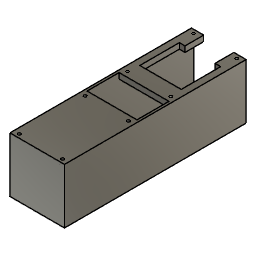
6_Cell_Lipo_Holder v3 (Autodesk Fusion 360 design; units mm, degrees)
Autodesk Fusion 360 part; units mm, degrees
sketch "Sketch1" plane through (0, 0, 0) normal (0, 1, 0) x (1, 0, 0)
  line L0 (26, -24.75) -> (-26, -24.75)
  line L1 (-26, -24.75) -> (-26, 24.75)
  line L2 (-26, 24.75) -> (26, 24.75)
  line L3 (26, 24.75) -> (26, -24.75)
  line L4 (26, -24.75) -> (-26, 24.75) construction
  line L5 (-26, -24.75) -> (26, 24.75) construction
  dimension "d1" = 52
  dimension "d2" = 49.5
  constraint horizontal L0
  constraint perpendicular L0 L1
  constraint parallel L0 L2
  constraint parallel L1 L3
  constraint coincident L4 origin
  constraint coincident L5 origin
  measures "d1" distance of L0.start L0.end
  measures "d2" distance of L0.start L2.end
extrude "Extrude1" add sketch "Sketch1" along normal blind 155 makes body 1
sketch "Sketch2" plane through (0, 0, 0) normal (0, -1, 0) x (1, 0, 0)
  line L0 (-26, -24.75) -> (26, -24.75)
  line L1 (26, -24.75) -> (26, 24.75)
  line L2 (26, 24.75) -> (-26, 24.75)
  line L3 (-26, 24.75) -> (-26, -24.75)
  line L4 (32, 30.75) -> (-32, 30.75)
  line L5 (-32, 30.75) -> (-32, -30.75)
  line L6 (-32, -30.75) -> (32, -30.75)
  line L7 (32, -30.75) -> (32, 30.75)
  line L8 (32, 30.75) -> (-32, -30.75) construction
  line L9 (-32, 30.75) -> (32, -30.75) construction
  dimension "d5" = 64
  dimension "d6" = 61.5
  constraint horizontal L4
  constraint perpendicular L4 L5
  constraint parallel L4 L6
  constraint parallel L5 L7
  constraint coincident L8 origin
  constraint coincident L9 origin
  measures "d5" distance of L4.start L4.end
  measures "d6" distance of L4.start L6.end
extrude "Extrude2" add sketch "Sketch2" against normal blind 193 separate body contours L0 L1 L2 L3 | L4 L5 L6 L7 makes body 2
sketch "Sketch3" plane through (0, 193, 0) normal (0, 1, 0) x (-1, 0, 0)
  line L0 (-32, 30.75) -> (-32, -30.75)
  line L1 (-32, -30.75) -> (32, -30.75)
  line L2 (32, -30.75) -> (32, 30.75)
  line L3 (32, 30.75) -> (-32, 30.75)
  line L4 (26, 24.75) -> (-26, 24.75)
  line L5 (-26, 24.75) -> (-26, -24.75)
  line L6 (-26, -24.75) -> (26, -24.75)
  line L7 (26, -24.75) -> (26, 24.75)
  line L8 (26, 24.75) -> (-26, -24.75) construction
  line L9 (-26, 24.75) -> (26, -24.75) construction
  dimension "d9" = 52
  dimension "d10" = 49.5
  constraint horizontal L4
  constraint perpendicular L4 L5
  constraint parallel L4 L6
  constraint parallel L5 L7
  constraint coincident L8 origin
  constraint coincident L9 origin
  measures "d9" distance of L4.start L4.end
  measures "d10" distance of L4.start L6.end
extrude "Extrude3" cut sketch "Sketch3" against normal blind 160 contours L4 L5 L6 L7 bodies 2
move_body "Move1" bodies 1 to x (1, 0, 0) y (0, 1, 0) z (0, 0, 1) at (0, 320, 0)
sketch "Sketch6" plane through (0, 0, 30.75) normal (0, 0, 1) x (-1, 0, 0)
  line L0 (32, 0) -> (-32, 0)
  line L1 (-32, 0) -> (-32, -193)
  line L2 (-32, -193) -> (32, -193)
  line L3 (32, -193) -> (32, 0)
  line L4 (0, 0) -> (0, -193)
  line L5 (32, -96.5) -> (-32, -96.5)
  circle A0 centre (-23, -4) radius 1.5
  circle A1 centre (23, -4) radius 1.5
  circle A2 centre (-23, -74) radius 1.5
  circle A3 centre (23, -74) radius 1.5
  circle A4 centre (-23, -119) radius 1.5
  circle A5 centre (23, -119) radius 1.5
  circle A6 centre (23, -189) radius 1.5
  circle A7 centre (-23, -189) radius 1.5
  line L6 (26, -79.5) -> (-26, -79.5)
  line L7 (-26, -79.5) -> (-26, -113.5)
  line L8 (-26, -113.5) -> (26, -113.5)
  line L9 (26, -113.5) -> (26, -79.5)
  line L10 (26, -79.5) -> (-26, -113.5) construction
  line L11 (-26, -79.5) -> (26, -113.5) construction
  line L12 (22, -131.0349) -> (-22, -131.0349)
  line L13 (-22, -131.0349) -> (-22, -173.0349)
  line L14 (-22, -173.0349) -> (22, -173.0349)
  line L15 (22, -173.0349) -> (22, -131.0349)
  line L16 (22, -131.0349) -> (-22, -173.0349) construction
  line L17 (-22, -131.0349) -> (22, -173.0349) construction
  point P0 (0, -96.5)
  point P1 (0, -152.0349)
  dimension "d45" = 3
  dimension "d46" = 3
  dimension "d47" = 3
  dimension "d48" = 3
  dimension "d49" = 3
  dimension "d50" = 3
  dimension "d51" = 3
  dimension "d52" = 3
  dimension "d53" = 23
  dimension "d54" = 23
  dimension "d55" = 23
  dimension "d56" = 23
  dimension "d57" = 22.5
  dimension "d58" = 22.5
  dimension "d59" = 70
  dimension "d60" = 70
  dimension "d89" = 52
  dimension "d90" = 34
  dimension "d101" = 44
  dimension "d102" = 42
  constraint coincident L4.start origin
  constraint midpoint L2 L4.end
  constraint midpoint L3 L5.start
  constraint midpoint L1 L5.end
  constraint symmetric L4 A0.centre A1.centre
  constraint symmetric L4 A2.centre A3.centre
  constraint symmetric L4 A4.centre A5.centre
  constraint symmetric L4 A6.centre A7.centre
  constraint horizontal L6
  constraint perpendicular L6 L7
  constraint parallel L6 L8
  constraint parallel L7 L9
  constraint coincident L10 P0
  constraint coincident L11 P0
  constraint midpoint L5 P0
  constraint horizontal L12
  constraint perpendicular L12 L13
  constraint parallel L12 L14
  constraint parallel L13 L15
  constraint coincident L16 P1
  constraint coincident L17 P1
  constraint coincident L4 P1
  measures "d45" diameter of A0
  measures "d46" diameter of A1
  measures "d47" diameter of A2
  measures "d48" diameter of A3
  measures "d49" diameter of A5
  measures "d50" diameter of A4
  measures "d51" diameter of A7
  measures "d52" diameter of A6
  measures "d53" distance of L4 A0.centre
  measures "d54" distance of L4 A2.centre
  measures "d55" distance of L4 A4.centre
  measures "d56" distance of L4 A7.centre
  measures "d57" distance of L5 A2.centre
  measures "d58" distance of L5 A4.centre
  measures "d59" distance of A0.centre A2.centre
  measures "d60" distance of A4.centre A7.centre
  measures "d89" distance of L6.start L6.end
  measures "d90" distance of L6.end L7.end
  measures "d101" distance of L12.start L12.end
  measures "d102" distance of L12.end L13.end
extrude "Extrude4" cut sketch "Sketch6" against normal blind 80 contours A0 | A1 | A2 | A3 | A4 | A5 | A6 | A7 bodies 2
sketch "Sketch7" plane through (0, 0, -30.75) normal (0, 0, -1) x (1, 0, 0)
  circle A0 centre (-23, -119) radius 1.5
  circle A1 centre (-23, -4) radius 1.5
  circle A2 centre (-23, -74) radius 1.5
  circle A3 centre (-23, -189) radius 1.5
  circle A4 centre (23, -119) radius 1.5
  circle A5 centre (23, -4) radius 1.5
  circle A6 centre (23, -74) radius 1.5
  circle A7 centre (23, -189) radius 1.5
  line L0 (32, 0) -> (-32, 0)
  line L1 (-32, 0) -> (-32, -193)
  line L2 (-32, -193) -> (32, -193)
  line L3 (32, -193) -> (32, 0)
  line L4 (20, -6) -> (26, -6)
  line L5 (26, -6) -> (26, -2)
  line L6 (26, -2) -> (20, -2)
  line L7 (20, -2) -> (20, -6)
  line L8 (20, -6) -> (26, -2) construction
  line L9 (26, -6) -> (20, -2) construction
  line L10 (-26, -6) -> (-20, -6)
  line L11 (-20, -6) -> (-20, -2)
  line L12 (-20, -2) -> (-26, -2)
  line L13 (-26, -2) -> (-26, -6)
  line L14 (-26, -6) -> (-20, -2) construction
  line L15 (-20, -6) -> (-26, -2) construction
  line L16 (20, -76) -> (26, -76)
  line L17 (26, -76) -> (26, -72)
  line L18 (26, -72) -> (20, -72)
  line L19 (20, -72) -> (20, -76)
  line L20 (20, -76) -> (26, -72) construction
  line L21 (26, -76) -> (20, -72) construction
  line L22 (-26, -76) -> (-20, -76)
  line L23 (-20, -76) -> (-20, -72)
  line L24 (-20, -72) -> (-26, -72)
  line L25 (-26, -72) -> (-26, -76)
  line L26 (-26, -76) -> (-20, -72) construction
  line L27 (-20, -76) -> (-26, -72) construction
  line L28 (-26, -121) -> (-20, -121)
  line L29 (-20, -121) -> (-20, -117)
  line L30 (-20, -117) -> (-26, -117)
  line L31 (-26, -117) -> (-26, -121)
  line L32 (-26, -121) -> (-20, -117) construction
  line L33 (-20, -121) -> (-26, -117) construction
  line L34 (20, -121) -> (26, -121)
  line L35 (26, -121) -> (26, -117)
  line L36 (26, -117) -> (20, -117)
  line L37 (20, -117) -> (20, -121)
  line L38 (20, -121) -> (26, -117) construction
  line L39 (26, -121) -> (20, -117) construction
  line L40 (20, -191) -> (26, -191)
  line L41 (26, -191) -> (26, -187)
  line L42 (26, -187) -> (20, -187)
  line L43 (20, -187) -> (20, -191)
  line L44 (20, -191) -> (26, -187) construction
  line L45 (26, -191) -> (20, -187) construction
  line L46 (-26, -191) -> (-20, -191)
  line L47 (-20, -191) -> (-20, -187)
  line L48 (-20, -187) -> (-26, -187)
  line L49 (-26, -187) -> (-26, -191)
  line L50 (-26, -191) -> (-20, -187) construction
  line L51 (-20, -191) -> (-26, -187) construction
  point P0 (23, -4)
  point P1 (-23, -4)
  point P2 (23, -74)
  point P3 (-23, -74)
  point P4 (-23, -119)
  point P5 (23, -119)
  point P6 (23, -189)
  point P7 (-23, -189)
  dimension "d63" = 6
  dimension "d64" = 4
  constraint horizontal L4
  constraint perpendicular L4 L5
  constraint parallel L4 L6
  constraint parallel L5 L7
  constraint coincident L8 P0
  constraint coincident L9 P0
  constraint coincident P0 A5.centre
  constraint horizontal L10
  constraint perpendicular L10 L11
  constraint parallel L10 L12
  constraint parallel L11 L13
  constraint coincident L14 P1
  constraint coincident L15 P1
  constraint coincident P1 A1.centre
  constraint horizontal L16
  constraint perpendicular L16 L17
  constraint parallel L16 L18
  constraint parallel L17 L19
  constraint coincident L20 P2
  constraint coincident L21 P2
  constraint coincident P2 A6.centre
  constraint horizontal L22
  constraint perpendicular L22 L23
  constraint parallel L22 L24
  constraint parallel L23 L25
  constraint coincident L26 P3
  constraint coincident L27 P3
  constraint coincident A2.centre P3
  constraint horizontal L28
  constraint perpendicular L28 L29
  constraint parallel L28 L30
  constraint parallel L29 L31
  constraint coincident L32 P4
  constraint coincident L33 P4
  constraint coincident P4 A0.centre
  constraint horizontal L34
  constraint perpendicular L34 L35
  constraint parallel L34 L36
  constraint parallel L35 L37
  constraint coincident L38 P5
  constraint coincident L39 P5
  constraint coincident A4.centre P5
  constraint horizontal L40
  constraint perpendicular L40 L41
  constraint parallel L40 L42
  constraint parallel L41 L43
  constraint coincident L44 P6
  constraint coincident L45 P6
  constraint coincident P6 A7.centre
  constraint horizontal L46
  constraint perpendicular L46 L47
  constraint parallel L46 L48
  constraint parallel L47 L49
  constraint coincident L50 P7
  constraint coincident L51 P7
  constraint coincident P7 A3.centre
  measures "d63" distance of L4.start L4.end
  measures "d64" distance of L4.end L5.end
extrude "Extrude5" cut sketch "Sketch7" against normal blind 20 contours L4 L5 L6 L7 | L10 L11 L12 L13 | L16 L17 L18 L19 | L22 L23 L24 L25 | L28 L29 L30 L31 | L34 L35 L36 L37 | L40 L41 L42 L43 | L46 L47 L48 L49 bodies 2
sketch "Sketch8" plane through (0, 0, 24.75) normal (0, 0, -1) x (1, 0, 0)
  circle A0 centre (-23, -119) radius 1.5
  circle A1 centre (-23, -74) radius 1.5
  circle A2 centre (-23, -189) radius 1.5
  circle A3 centre (23, -119) radius 1.5
  circle A4 centre (23, -74) radius 1.5
  circle A5 centre (23, -189) radius 1.5
  line L0 (-26, -193) -> (26, -193)
  line L1 (26, -193) -> (26, -33)
  line L2 (26, -33) -> (-26, -33)
  line L3 (-26, -33) -> (-26, -193)
  circle A6 centre (23, -189) radius 2.9
  circle A7 centre (-23, -189) radius 2.9
  circle A8 centre (-23, -119) radius 2.9
  circle A9 centre (23, -119) radius 2.9
  circle A10 centre (23, -74) radius 2.9
  circle A11 centre (-23, -74) radius 2.9
  circle A12 centre (23, -4.0001) radius 2.9
  circle A13 centre (-23, -4.0001) radius 2.9
  dimension "d67" = 5.8
  dimension "d68" = 5.8
  dimension "d69" = 5.8
  dimension "d70" = 5.8
  dimension "d71" = 5.8
  dimension "d72" = 5.8
  dimension "d73" = 5.8
  dimension "d74" = 5.8
  constraint concentric A5 A6
  constraint concentric A2 A7
  constraint concentric A0 A8
  constraint concentric A3 A9
  constraint concentric A4 A10
  constraint concentric A1 A11
  measures "d67" diameter of A6
  measures "d68" diameter of A7
  measures "d69" diameter of A9
  measures "d70" diameter of A8
  measures "d71" diameter of A10
  measures "d72" diameter of A11
  measures "d73" diameter of A12
  measures "d74" diameter of A13
extrude "Extrude6" cut sketch "Sketch8" against normal blind 2.3 contours A6 | A7 | A8 | A9 | A10 | A11 | A12 | A13 bodies 2
extrude "Extrude7" cut 1 faces at (32, 64.3333, -10.25) along direction (-1, 0, 0) blind 3 on bodies 2 bodies 2
extrude "Extrude8" cut 1 faces at (-32, 64.3333, 10.25) along direction (1, 0, 0) blind 3 on bodies 2 bodies 2
extrude "Extrude9" cut 1 faces at (6.6667, 50, -30.75) along direction (0, 0, 1) blind 3 on bodies 2 bodies 2
extrude "Extrude10" cut 1 faces at (26, 114.3333, 8.25) along direction (1, 0, 0) blind 0.5 on bodies 2 bodies 2
extrude "Extrude11" cut 1 faces at (-26, 114.3333, 8.25) along direction (-1, 0, 0) blind 0.5 on bodies 2 bodies 2
extrude "Extrude12" cut 1 faces at (-6.6667, 165, -24.75) along direction (0, 0, -1) blind 0.5 on bodies 2 bodies 2
extrude "Extrude13" cut sketch "Sketch6" against normal blind 10 contours L4 L5 L6 L9 | L4 L5 L6 L7 | L4 L5 L8 L9 | L4 L5 L7 L8 bodies 2
extrude "Extrude14" cut 1 faces at (-26, 90.8333, 26.75) along direction (-1, 0, 0) blind 0.5 on bodies 2 bodies 2
extrude "Extrude15" cut 1 faces at (26, 102.1667, 26.75) along direction (1, 0, 0) blind 0.5 on bodies 2 bodies 2
sketch "Sketch9" plane through (0, 193, 0) normal (0, 1, 0) x (-1, 0, 0)
  line L0 (-26.5, -25.25) -> (-26.5, 24.75)
  line L1 (-26.5, 24.75) -> (26.5, 24.75)
  line L2 (26.5, 24.75) -> (26.5, -25.25)
  line L3 (26.5, -25.25) -> (-26.5, -25.25)
  line L4 (-29, -27.75) -> (29, -27.75)
  line L5 (29, -27.75) -> (29, 30.75)
  line L6 (29, 30.75) -> (-29, 30.75)
  line L7 (-29, 30.75) -> (-29, -27.75)
  line L8 (-22, 30.75) -> (-22, 24.75)
  line L9 (22, 30.75) -> (22, 24.75)
  line L10 (0, 0) -> (0, 30.75)
  line L11 (-16, 30.75) -> (-16, 24.75)
  line L12 (16, 30.75) -> (16, 24.75)
  dimension "d97" = 22
  dimension "d98" = 22
  dimension "d99" = 6
  dimension "d100" = 6
  constraint coincident L6 L8.start
  constraint coincident L1 L8.end
  constraint perpendicular L1 L8
  constraint coincident L6 L9.start
  constraint coincident L1 L9.end
  constraint perpendicular L1 L9
  constraint coincident L10.start origin
  constraint midpoint L6 L10.end
  constraint coincident L6 L11.start
  constraint coincident L1 L11.end
  constraint perpendicular L1 L11
  constraint coincident L6 L12.start
  constraint coincident L1 L12.end
  constraint perpendicular L6 L12
  measures "d97" distance of L8 L10
  measures "d98" distance of L9 L10
  measures "d99" distance of L8 L11
  measures "d100" distance of L9 L12
extrude "Extrude16" cut sketch "Sketch6" against normal blind 8 contours L4 L12 L13 L14 | L4 L12 L14 L15 bodies 2
extrude "Extrude17" cut sketch "Sketch9" against normal blind 28 contours L1 L6 L10 L11 | L1 L6 L10 L12 bodies 2
extrude "Extrude18" cut 2 faces at (-20.5, 4, -10.75) (20.5, 4, -10.75) along direction (0, 0, 1) blind 40 on bodies 2 bodies 2
extrude "Extrude19" cut 1 faces at (8.8333, 33, 8.0833) along direction (0, -1, 0) blind 16.5 on bodies 2 bodies 2
extrude "Extrude20" add 1 faces at (-25.5, 4, 29.25) along direction (0, 0, -1) blind 1.2 on bodies 2 bodies 2
extrude "Extrude21" add 1 faces at (-25.5, 4, 28.05) along direction (0, 0, -1) blind 1 on bodies 2 bodies 2
extrude "Extrude22" add 1 faces at (20.5, 4, 29.25) along direction (0, 0, -1) blind 2.2 on bodies 2 bodies 2
move_body "Move2" bodies 1 to x (1, 0, 0) y (0, 1, 0) z (0, 0, 1) at (0, -100, 0)
sketch "Sketch10" plane through (0, 16.5, 0) normal (0, 1, 0) x (-1, 0, 0)
  line L0 (26.5, 24.75) -> (-26.5, 24.75)
  line L1 (-26.5, 24.75) -> (-26.5, -25.25)
  line L2 (-26.5, -25.25) -> (26.5, -25.25)
  line L3 (26.5, -25.25) -> (26.5, 24.75)
  line L4 (20, 20) -> (-20, 20)
  line L5 (-20, 20) -> (-20, -20)
  line L6 (-20, -20) -> (20, -20)
  line L7 (20, -20) -> (20, 20)
  line L8 (20, 20) -> (-20, -20) construction
  line L9 (-20, 20) -> (20, -20) construction
  constraint horizontal L4
  constraint perpendicular L4 L5
  constraint parallel L4 L6
  constraint parallel L5 L7
  constraint coincident L8 origin
  constraint coincident L9 origin
extrude "Extrude23" cut sketch "Sketch10" against normal blind 14.5 contours L4 L5 L6 L7 bodies 2
hidden bodies 1
